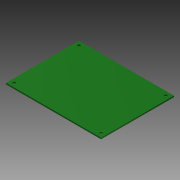
# Autodesk Inventor part: pcb
Saved by Autodesk Inventor 2013 (Build 170138000, 138)
## iProperties
Created: 2013-04-17
Part Number: pcb
Material: Résine phénolique
Document SubType Name: Modeling
Designer: dimercur
Density: 1.38 g/cm^3
Mass: 22.7954 g
Surface Area: 213.04 cm^2
Volume: 16.5184 cm^3
Author: dimercur
Autodesk Inventor part; units mm, degrees
ref_plane "YZ Plane" through (0, 0, 0) normal (1, 0, 0) x (0, 1, 0)
ref_plane "XZ Plane" through (0, 0, 0) normal (0, 1, 0) x (-1, 0, 0)
ref_plane "XY Plane" through (0, 0, 0) normal (0, 0, 1) x (1, 0, 0)
sketch "Esquisse1" plane through (0, 0, 0) normal (0, 0, 1) x (1, 0, 0)
  line L0 (51.6387, -29.6903) -> (-64.3613, -29.6903)
  line L1 (-64.3613, -29.6903) -> (-64.3613, 59.3097)
  line L2 (-64.3613, 59.3097) -> (51.6387, 59.3097)
  line L3 (51.6387, 59.3097) -> (51.6387, -29.6903)
  point P0 (0, 0)
  dimension "d0" = 116
  dimension "d2" = 89
  constraints: 8 end point, 2 parallel, 1 horizontal, 1 perpendicular
  measures "d0" distance of L1.end L2.end
  measures "d2" distance of L0.end L1.end
extrude "Extrusion1" add sketch "Esquisse1" along normal blind 1.6
sketch "Esquisse2" plane through (0, 0, 1.6) normal (0, 0, 1) x (1, 0, 0)
  line L0 (-64.3613, -29.6903) -> (51.6387, -29.6903) projected
  line L1 (51.6387, 59.3097) -> (-64.3613, 59.3097) projected
  line L2 (-64.3613, 59.3097) -> (-64.3613, -29.6903) projected
  circle A0 centre (-59.3613, 54.3097) radius 1.6
  circle A1 centre (-59.3613, -24.6903) radius 1.6
  circle A2 centre (46.6387, -24.6903) radius 1.6
  circle A3 centre (46.6387, 54.3097) radius 1.6
  point P0 (0, 0)
  dimension "d5" = 3.2
  dimension "d7" = 3.2
  dimension "d8" = 3.2
  dimension "d9" = 3.2
  dimension "d10" = 79
  dimension "d11" = 79
  dimension "d12" = 5
  dimension "d13" = 5
  dimension "d14" = 106
  dimension "d15" = 106
  dimension "d16" = 5
  dimension "d17" = 5
  constraints: 4 centre point
  measures "d5" diameter of A0
  measures "d7" diameter of A3
  measures "d8" diameter of A1
  measures "d9" diameter of A2
  measures "d10" distance of A2.centre A3.centre
  measures "d11" distance of A1.centre A0.centre
  measures "d12" distance from line of L0 A1.centre
  measures "d13" distance from line of L1 A3.centre
  measures "d14" distance of A3.centre A0.centre
  measures "d15" distance of A2.centre A1.centre
  measures "d16" distance from line of L2 A0.centre
  measures "d17" distance from line of L2 A1.centre
extrude "Extrusion2" cut sketch "Esquisse2" against normal blind 1.6
